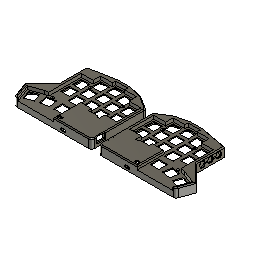
top_23332_3 (Autodesk Fusion 360 design; units mm, degrees)
Autodesk Fusion 360 part; units mm, degrees
sketch "case_plate_23332_3" plane through (0, 0, 0) normal (0, 0, 1) x (1, 0, 0)
  line L0 (107.5, 54.6647) -> (107.5, 98.826)
  line L1 (28.1017, 101.4312) -> (8.5, 89.0512)
  line L2 (107.5, 98.826) -> (67.6888, 106.482)
  line L3 (8.5, 89.0512) -> (8.5, 7.28)
  line L4 (67.5953, 106.5) -> (48.3769, 106.5)
  line L5 (126.2948, 7.28) -> (133.9348, 28.2707)
  line L6 (8.5, 7.28) -> (126.2948, 7.28)
  line L7 (67.6888, 106.482) -> (67.5953, 106.5)
  line L8 (48.3769, 106.5) -> (28.1017, 101.4312)
  line L9 (133.9348, 28.2707) -> (107.5, 54.6647)
  line L10 (48.0076, 109.5) -> (26.9069, 104.2248)
  line L11 (110.5, 101.3041) -> (67.8811, 109.5)
  line L12 (5.5, 90.7047) -> (5.5, 4.28)
  line L13 (128.3954, 4.28) -> (137.4081, 29.0421)
  line L14 (137.4081, 29.0421) -> (110.5, 55.9087)
  line L15 (5.5, 4.28) -> (128.3954, 4.28)
  line L16 (67.8811, 109.5) -> (48.0076, 109.5)
  line L17 (110.5, 55.9087) -> (110.5, 101.3041)
  line L18 (26.9069, 104.2248) -> (5.5, 90.7047)
  line L19 (67.7096, 107.7) -> (48.2292, 107.7)
  line L20 (27.6238, 102.5487) -> (7.3, 89.7126)
  line L21 (108.7, 55.1623) -> (108.7, 99.8172)
  line L22 (135.3241, 28.5793) -> (108.7, 55.1623)
  line L23 (7.3, 89.7126) -> (7.3, 6.08)
  line L24 (7.3, 6.08) -> (127.135, 6.08)
  line L25 (48.2292, 107.7) -> (27.6238, 102.5487)
  line L26 (127.135, 6.08) -> (135.3241, 28.5793)
  line L27 (108.7, 99.8172) -> (67.7096, 107.7)
  line L28 (68.0288, 108.2496) -> (67.7668, 108.3)
  line L29 (67.7668, 108.3) -> (48.1553, 108.3)
  line L30 (27.3848, 103.1074) -> (6.7, 90.0433)
  line L31 (6.7, 90.0433) -> (6.7, 5.48)
  line L32 (109.3, 55.4111) -> (109.3, 100.3128)
  line L33 (48.1553, 108.3) -> (27.3848, 103.1074)
  line L34 (136.0188, 28.7336) -> (109.3, 55.4111)
  line L35 (6.7, 5.48) -> (127.5552, 5.48)
  line L36 (127.5552, 5.48) -> (136.0188, 28.7336)
  line L37 (109.3, 100.3128) -> (68.0288, 108.2496)
  circle A0 centre (32, 80.5) radius 2.2
  circle A1 centre (84, 80.5) radius 2.2
  circle A2 centre (100.1356, 36.6759) radius 2.2
  line L38 (10.5, 10.39) -> (43.5, 10.39)
  line L39 (43.5, 28.39) -> (10.5, 28.39)
  line L40 (43.5, 10.39) -> (43.5, 28.39)
  line L41 (10.5, 28.39) -> (10.5, 10.39)
  line L42 (47.025, 13.01) -> (47.025, 7.16)
  line L43 (55.825, 7.16) -> (55.825, 13.01)
  line L44 (55.825, 13.01) -> (47.025, 13.01)
  line L45 (66.825, 12.025) -> (57.825, 12.025)
  line L46 (57.825, 12.025) -> (57.825, 8.525)
  line L47 (57.825, 8.525) -> (66.825, 8.525)
  line L48 (66.825, 8.525) -> (66.825, 12.025)
  line L49 (122.6064, 37.8282) -> (114.8282, 45.6064)
  line L50 (114.8282, 45.6064) -> (108.3936, 39.1718)
  line L51 (108.3936, 39.1718) -> (110.7259, 36.8394)
  line L52 (118.9049, 34.1268) -> (122.6064, 37.8282)
  line L53 (43.2, 31.55) -> (43.2, 40.45)
  line L54 (43.2, 40.45) -> (35.1996, 40.45)
  line L55 (34.6, 39.7287) -> (34.6, 31.55)
  line L56 (34.6, 31.55) -> (43.2, 31.55)
  line L57 (27, 52) -> (27, 66)
  line L58 (13, 52) -> (27, 52)
  line L59 (13, 66) -> (13, 52)
  line L60 (27, 66) -> (13, 66)
  line L61 (27, 71) -> (27, 85)
  line L62 (13, 85) -> (13, 71)
  line L63 (13, 71) -> (27, 71)
  line L64 (27, 85) -> (13, 85)
  line L65 (46, 59) -> (32, 59)
  line L66 (46, 45) -> (46, 59)
  line L67 (32, 45) -> (46, 45)
  line L68 (32, 59) -> (32, 45)
  line L69 (32, 78) -> (32, 64)
  line L70 (46, 64) -> (46, 78)
  line L71 (32, 64) -> (46, 64)
  line L72 (46, 78) -> (32, 78)
  line L73 (46, 97) -> (32, 97)
  line L74 (32, 83) -> (46, 83)
  line L75 (46, 83) -> (46, 97)
  line L76 (32, 97) -> (32, 83)
  line L77 (51, 64) -> (51, 50)
  line L78 (51, 50) -> (65, 50)
  line L79 (65, 50) -> (65, 64)
  line L80 (65, 64) -> (51, 64)
  line L81 (65, 69) -> (65, 83)
  line L82 (65, 83) -> (51, 83)
  line L83 (51, 83) -> (51, 69)
  line L84 (51, 69) -> (65, 69)
  line L85 (65, 102) -> (51, 102)
  line L86 (51, 102) -> (51, 88)
  line L87 (65, 88) -> (65, 102)
  line L88 (51, 88) -> (65, 88)
  line L89 (84, 59) -> (70, 59)
  line L90 (70, 59) -> (70, 45)
  line L91 (70, 45) -> (84, 45)
  line L92 (84, 45) -> (84, 59)
  line L93 (84, 64) -> (84, 78)
  line L94 (70, 78) -> (70, 64)
  line L95 (84, 78) -> (70, 78)
  line L96 (70, 64) -> (84, 64)
  line L97 (70, 83) -> (84, 83)
  line L98 (70, 97) -> (70, 83)
  line L99 (84, 83) -> (84, 97)
  line L100 (84, 97) -> (70, 97)
  line L101 (89, 66) -> (89, 52)
  line L102 (103, 52) -> (103, 66)
  line L103 (103, 66) -> (89, 66)
  line L104 (89, 52) -> (103, 52)
  line L105 (103, 85) -> (89, 85)
  line L106 (103, 71) -> (103, 85)
  line L107 (89, 85) -> (89, 71)
  line L108 (89, 71) -> (103, 71)
  line L109 (70, 36.2) -> (70, 22.2)
  line L110 (84, 36.2) -> (70, 36.2)
  line L111 (70, 22.2) -> (84, 22.2)
  line L112 (84, 22.2) -> (84, 36.2)
  line L113 (104.164, 19.211) -> (106.5951, 32.9983)
  line L114 (106.5951, 32.9983) -> (92.8078, 35.4294)
  line L115 (92.8078, 35.4294) -> (90.3767, 21.6421)
  line L116 (90.3767, 21.6421) -> (104.164, 19.211)
  line L117 (110.347, 17.5543) -> (123.5027, 12.766)
  line L118 (115.1353, 30.71) -> (110.347, 17.5543)
  line L119 (123.5027, 12.766) -> (128.291, 25.9217)
  line L120 (128.291, 25.9217) -> (115.1353, 30.71)
  line L121 (8.5, 49.25) -> (29.25, 49.25)
  line L122 (10.25, 49.25) -> (10.25, 87.75)
  line L123 (29.25, 87.75) -> (10.25, 87.75)
  line L124 (48.75, 42.25) -> (48.75, 47.25)
  line L125 (29.25, 49.25) -> (29.25, 42.25)
  line L126 (48.25, 99.75) -> (29.25, 99.75)
  line L127 (29.25, 99.75) -> (29.25, 87.75)
  line L128 (48.75, 47.25) -> (67.25, 47.25)
  line L129 (67.75, 99.75) -> (67.75, 104.75)
  line L130 (67.75, 104.75) -> (48.25, 104.75)
  line L131 (48.25, 104.75) -> (48.25, 99.75)
  line L132 (67.25, 4.28) -> (67.25, 47.25)
  line L133 (86.75, 87.75) -> (86.75, 99.75)
  line L134 (86.75, 99.75) -> (67.75, 99.75)
  line L135 (105.75, 54.6647) -> (105.75, 87.75)
  line L136 (105.75, 87.75) -> (86.75, 87.75)
  line L137 (67.25, 19.45) -> (86.9722, 19.45)
  line L138 (86.9722, 19.45) -> (106.6135, 15.9867)
  line L139 (105.75, 35.9398) -> (111.608, 34.9069)
  line L140 (106.6135, 15.9867) -> (125.1463, 9.2413)
  line L141 (123.3406, 4.28) -> (131.8157, 27.5653)
  line L142 (111.7483, 34.8693) -> (133.4723, 26.9624)
  line L143 (105.75, 54.6647) -> (107.5, 54.6647)
  line L144 (111.7483, 34.8693) -> (111.608, 34.9069)
  arc A3 (32, 40.3) -> (34.1857, 42.25) centre (32, 42.5) ccw
  line L145 (34.1857, 42.25) -> (48.75, 42.25)
  line L146 (32, 40.3) -> (29.25, 40.3)
  line L147 (29.25, 42.25) -> (29.25, 40.3)
  line L148 (105.75, 35.9398) -> (105.75, 54.6647)
  line L149 (107.5, 37.4082) -> (107.5, 54.6647)
  line L150 (107.5, 37.4082) -> (111.9871, 36.617)
  line L151 (112.275, 36.5399) -> (111.9871, 36.617)
  line L152 (112.275, 36.5399) -> (133.327, 28.8776)
  line L153 (8.5, 47.65) -> (27.65, 47.65)
  line L154 (27.65, 47.65) -> (27.65, 42.25)
  line L155 (27.65, 42.25) -> (27.65, 38.7)
  line L156 (32, 38.7) -> (27.65, 38.7)
  arc A4 (32, 38.7) -> (35.3193, 40.65) centre (32, 42.5) ccw
  line L157 (35.3193, 40.65) -> (50.35, 40.65)
  line L158 (50.35, 40.65) -> (50.35, 45.65)
  line L159 (50.35, 45.65) -> (65.65, 45.65)
  line L160 (65.65, 4.28) -> (65.65, 45.65)
extrude "Extrude1" add sketch "case_plate_23332_3" against normal blind 7.6 contours L15 L35 L132 L141 | L10 L11 L12 L13 L14 L15 L16 L17 L18 L28 L29 L30 L31 L32 L33 L34 L35 L36 L37 L141 L160 | L15 L35 L132 L160 makes body 1
extrude "Extrude2" add sketch "case_plate_23332_3" against normal blind 6.8 contours L0 L1 L2 L3 L4 L5 L6 L7 L8 L9 L19 L20 L21 L22 L23 L24 L25 L26 L27 L141 L160 | L6 L24 L132 L141 | L6 L24 L132 L160 | L24 L35 L132 L141 | L19 L20 L21 L22 L23 L24 L25 L26 L27 L28 L29 L30 L31 L32 L33 L34 L35 L36 L37 L141 L160 | L24 L35 L132 L160 bodies 1
extrude "Extrude3" add sketch "case_plate_23332_3" along normal blind 7 contours L0 L1 L2 L3 L4 L7 L8 L121 L122 L123 L126 L127 L129 L130 L131 L133 L134 L135 L136 L143 | L0 L1 L2 L3 L4 L5 L6 L7 L8 L9 L19 L20 L21 L22 L23 L24 L25 L26 L27 L141 L160 | L5 L9 L139 L142 L143 L144 L148 L149 L150 L151 L152 | L5 L6 L141 L142 | L6 L24 L132 L160 | L3 L6 L45 L47 L48 L121 L124 L125 L128 L132 A3 L145 L146 L147 L153 L154 L155 L156 A4 L157 L158 L159 L160 | L19 L20 L21 L22 L23 L24 L25 L26 L27 L28 L29 L30 L31 L32 L33 L34 L35 L36 L37 L141 L160 | L24 L35 L132 L160 | L10 L11 L12 L13 L14 L15 L16 L17 L18 L28 L29 L30 L31 L32 L33 L34 L35 L36 L37 L141 L160 | L45 L47 L48 L160 | L15 L35 L132 L160 bodies 1
extrude "Extrude4" add sketch "case_plate_23332_3" along normal blind 1.6 contours L121 L122 L123 L124 L125 L126 L127 L128 L129 L130 L131 L132 L133 L134 L135 L136 L137 L138 L139 L140 L141 L142 L144 A3 L145 L146 L147 L148 | L6 L24 L132 L141 | L6 L132 L137 L138 L140 L141 | L24 L35 L132 L141 | L15 L35 L132 L141 | A0 | A1 | A2 bodies 1
extrude "Extrude5" add sketch "case_plate_23332_3" along normal blind 1.6 from surface at 5.4 contours L9 L49 L50 L51 L52 L149 L150 L152 | L49 L50 L51 L52 L150 L151 L152 | L3 L6 L42 L43 L44 L45 L46 L47 L53 L54 L55 L56 L153 L154 L155 L156 A4 L157 L158 L159 L160 | L6 L42 L43 L44 | L45 L46 L47 L160 | L53 L54 L55 L56 A4 | L38 L39 L40 L41 bodies 1
move_body "Move1" bodies 1 to x (1, 0, 0) y (0, 1, 0) z (0, 0, 1) at (0, 0, -1.6)
hole "Hole1" at (32, 80.5, 0) at (32, 42.5, 0) at (84, 80.5, 0) at (100.1356, 36.6759, 0) direction (0, 0, -1) diameter 2.4 depth 10 tip angle 118 countersink diameter 4.4 countersink angle 90 bodies 1
sketch "Sketch2" plane through (5.5, 0, 0) normal (-1, 0, 0) x (0, -1, 0)
  line L0 (-90.7047, 5.4) -> (-90.7047, -9.2)
  line L1 (-90.7047, -9.2) -> (-4.28, -9.2)
  line L2 (-4.28, -9.2) -> (-4.28, 5.4)
  line L3 (-4.28, 5.4) -> (-90.7047, 5.4)
  line L4 (-28.39, 0) -> (-10.39, 0)
  line L5 (-30.3566, 4.2) -> (-8.4131, 4.2)
  line L6 (-30.3566, -3.8) -> (-7.9707, -3.8)
  line L7 (-25.39, 4.2) -> (-25.39, -3.8)
  line L8 (-13.39, 4.2) -> (-13.39, -3.8)
  dimension "d17" = 1.2
  dimension "d18" = 8
  dimension "d19" = 3
  dimension "d20" = 12
  constraint perpendicular L2 L5
  constraint horizontal L6
  constraint coincident L5 L7.start
  constraint coincident L6 L7.end
  constraint perpendicular L6 L7
  constraint coincident L5 L8.start
  constraint coincident L6 L8.end
  constraint perpendicular L6 L8
  measures "d17" distance of L3 L5
  measures "d18" distance of L5 L6
  measures "d19" distance of L4.start L7
  measures "d20" distance of L7 L8
extrude "Extrude6" cut sketch "Sketch2" against normal up to surface (3 mm away) contours L4 L5 L7 L8 | L4 L6 L7 L8 bodies 1
chamfer "Chamfer2" distance 1 angle 45 4 edges at (5.5, 19.39, 4.2) (5.5, 25.39, 0.2) (5.5, 19.39, -3.8) (5.5, 13.39, 0.2) on bodies 1
sketch "Sketch3" plane through (0, 4.28, 0) normal (0, -1, 0) x (1, 0, 0)
  line L0 (5.5, 5.4) -> (5.5, -9.2)
  line L1 (5.5, -9.2) -> (128.3954, -9.2)
  line L2 (128.3954, -9.2) -> (128.3954, 5.4)
  line L3 (128.3954, 5.4) -> (123.3406, 5.4)
  line L4 (123.3406, 5.4) -> (123.3406, 0)
  line L5 (123.3406, 0) -> (67.25, 0)
  line L6 (67.25, 0) -> (67.25, 5.4)
  line L7 (67.25, 5.4) -> (5.5, 5.4)
  line L8 (55.825, 0) -> (47.025, 0)
  line L9 (46.3828, -5) -> (57.0469, -5) construction
  line L10 (46.1538, -4.25) -> (57.6357, -4.25) construction
  line L11 (49.425, 0) -> (49.425, -4.25) construction
  line L12 (53.425, 0) -> (53.425, -4.25) construction
  line L13 (49.425, -5.75) -> (53.425, -5.75)
  arc A0 (53.425, -5.75) -> (53.425, -2.75) centre (53.425, -4.25) ccw
  line L14 (53.425, -2.75) -> (49.425, -2.75)
  arc A1 (49.425, -2.75) -> (49.425, -5.75) centre (49.425, -4.25) ccw
  line L15 (49.425, -4.25) -> (53.425, -4.25) construction
  dimension "d23" = 10.4
  dimension "d24" = 0.75
  dimension "d25" = 2.4
  dimension "d26" = 4
  dimension "d27" = 3
  constraint horizontal L9
  constraint parallel L9 L10
  constraint coincident L8 L11.start
  constraint coincident L10 L11.end
  constraint perpendicular L10 L11
  constraint coincident L8 L12.start
  constraint coincident L10 L12.end
  constraint perpendicular L10 L12
  constraint tangent L13 A0
  constraint tangent A0 L14
  constraint parallel L13 L14
  constraint tangent L14 A1
  constraint tangent L13 A1
  constraint coincident L12.end A0.centre
  constraint perpendicular L12 L15
  constraint coincident L11.end A1.centre
  measures "d23" distance of L7 L9
  measures "d24" distance of L9 L10
  measures "d25" distance of L8.end L11
  measures "d26" distance of L11 L12
  measures "d27" diameter of A0
extrude "Extrude7" cut sketch "Sketch3" against normal up to surface (3 mm away) contours L13 A0 L14 A1 bodies 1
sketch "Sketch4" plane through (0, 0, -5.75) normal (0, 0, 1) x (-1, 0, 0)
  line L0 (-49.425, -4.28) -> (-53.425, -4.28)
  line L1 (-53.425, -4.28) -> (-53.425, -7.28)
  line L2 (-53.425, -7.28) -> (-49.425, -7.28)
  line L3 (-49.425, -7.28) -> (-49.425, -4.28)
  line L4 (-49.425, -5.78) -> (-53.425, -5.78)
  constraint midpoint L3 L4.start
  constraint midpoint L1 L4.end
extrude "Extrude8" cut sketch "Sketch4" against normal up to surface (2.65 mm away) contours L1 L2 L3 L4 bodies 1
chamfer "Chamfer1" distance 0.5 angle 45 4 edges at (51.425, 4.28, -2.75) (54.925, 4.28, -4.25) (51.425, 4.28, -5.75) (47.925, 4.28, -4.25) on bodies 1
sketch "Sketch5" plane through (83.1189, 83.2475, 0) normal (0.70656, 0.707653, 0) x (-0.707653, 0.70656, 0)
  line L0 (-76.7172, 5.4) -> (-76.7172, -9.2)
  line L1 (-76.7172, -9.2) -> (-38.6928, -9.2)
  line L2 (-38.6928, -9.2) -> (-38.6928, 5.4)
  line L3 (-38.6928, 5.4) -> (-76.7172, 5.4)
  line L4 (-76.7172, -5) -> (-38.6928, -5) construction
  line L5 (-60.0349, 0) -> (-49.0349, 0) construction
  line L6 (-58.0349, -3.1835) -> (-58.0349, -6.8453)
  line L7 (-51.0349, -3.1591) -> (-51.0349, -7.1366)
  line L8 (-58.0349, -4.5) -> (-51.0349, -4.5)
  line L9 (-58.0349, -5.5) -> (-51.0349, -5.5)
  dimension "d34" = 10.4
  dimension "d35" = 2
  dimension "d36" = 7
  dimension "d37" = 0.5
  dimension "d38" = 0.5
  constraint coincident L0 L4.start
  constraint coincident L2 L4.end
  constraint perpendicular L2 L4
  constraint perpendicular L4 L6
  constraint perpendicular L4 L7
  constraint coincident L6 L8.start
  constraint coincident L7 L8.end
  constraint perpendicular L7 L8
  constraint coincident L6 L9.start
  constraint coincident L7 L9.end
  constraint perpendicular L7 L9
  measures "d34" distance of L3 L4
  measures "d35" distance of L5.start L6
  measures "d36" distance of L6 L7
  measures "d37" distance of L4 L9
  measures "d38" distance of L4 L8
extrude "Extrude9" cut sketch "Sketch5" against normal up to surface (3 mm away) contours L6 L7 L8 L9 bodies 1
sketch "Sketch6" plane through (0, 0, 5.4) normal (0, 0, 1) x (-1, 0, 0)
  line L0 (-111.7483, -34.8693) -> (-131.8157, -27.5653)
  line L1 (-131.8157, -27.5653) -> (-123.3406, -4.28)
  line L2 (-123.3406, -4.28) -> (-128.3954, -4.28)
  line L3 (-128.3954, -4.28) -> (-137.4081, -29.0421)
  line L4 (-137.4081, -29.0421) -> (-110.5, -55.9087)
  line L5 (-110.5, -55.9087) -> (-110.5, -101.3041)
  line L6 (-110.5, -101.3041) -> (-67.8811, -109.5)
  line L7 (-67.8811, -109.5) -> (-48.0076, -109.5)
  line L8 (-48.0076, -109.5) -> (-26.9069, -104.2248)
  line L9 (-26.9069, -104.2248) -> (-5.5, -90.7047)
  line L10 (-5.5, -90.7047) -> (-5.5, -4.28)
  line L11 (-5.5, -4.28) -> (-67.25, -4.28)
  line L12 (-67.25, -4.28) -> (-67.25, -47.25)
  line L13 (-67.25, -47.25) -> (-48.75, -47.25)
  line L14 (-48.75, -47.25) -> (-48.75, -42.25)
  line L15 (-48.75, -42.25) -> (-34.1857, -42.25)
  arc A0 (-32, -40.3) -> (-34.1857, -42.25) centre (-32, -42.5) ccw
  line L16 (-32, -40.3) -> (-29.25, -40.3)
  line L17 (-29.25, -40.3) -> (-29.25, -49.25)
  line L18 (-29.25, -49.25) -> (-10.25, -49.25)
  line L19 (-10.25, -49.25) -> (-10.25, -87.75)
  line L20 (-10.25, -87.75) -> (-29.25, -87.75)
  line L21 (-29.25, -87.75) -> (-29.25, -99.75)
  line L22 (-29.25, -99.75) -> (-48.25, -99.75)
  line L23 (-48.25, -99.75) -> (-48.25, -104.75)
  line L24 (-48.25, -104.75) -> (-67.75, -104.75)
  line L25 (-67.75, -104.75) -> (-67.75, -99.75)
  line L26 (-67.75, -99.75) -> (-86.75, -99.75)
  line L27 (-86.75, -99.75) -> (-86.75, -87.75)
  line L28 (-86.75, -87.75) -> (-105.75, -87.75)
  line L29 (-105.75, -87.75) -> (-105.75, -35.9398)
  line L30 (-105.75, -35.9398) -> (-111.608, -34.9069)
  line L31 (-111.608, -34.9069) -> (-111.7483, -34.8693)
  line L32 (-66.825, -12.025) -> (-57.825, -12.025)
  line L33 (-57.825, -12.025) -> (-57.825, -8.525)
  line L34 (-57.825, -8.525) -> (-66.825, -8.525)
  line L35 (-66.825, -8.525) -> (-66.825, -12.025)
  line L36 (-59.325, -12.025) -> (-59.325, -8.525)
  line L37 (-65.325, -12.025) -> (-65.325, -8.525)
  dimension "d41" = 1.5
  dimension "d42" = 6
  constraint coincident L32 L36.start
  constraint coincident L34 L36.end
  constraint perpendicular L34 L36
  constraint coincident L32 L37.start
  constraint coincident L34 L37.end
  constraint perpendicular L34 L37
  measures "d41" distance of L33 L36
  measures "d42" distance of L36 L37
extrude "Extrude10" cut sketch "Sketch6" against normal up to surface (1.6 mm away) contours L32 L34 L36 L37 bodies 1
chamfer "Chamfer3" distance 0.4 angle 45 4 edges at (62.325, 12.025, 5.4) (59.325, 10.275, 5.4) (62.325, 8.525, 5.4) (65.325, 10.275, 5.4) on bodies 1
sketch "Sketch7" plane through (110.5, 0, 0) normal (1, 0, 0) x (0, 1, 0)
  line L0 (55.9087, 5.4) -> (55.9087, -9.2)
  line L1 (55.9087, -9.2) -> (101.3041, -9.2)
  line L2 (101.3041, -9.2) -> (101.3041, 5.4)
  line L3 (101.3041, 5.4) -> (55.9087, 5.4)
  line L4 (55.9087, -1.5) -> (101.3041, -1.5) construction
  line L5 (67.8782, 2.4883) -> (63.2884, 2.4616)
  line L6 (63.2884, 2.4616) -> (61.0165, -1.5266)
  line L7 (61.0165, -1.5266) -> (63.3345, -5.4883)
  line L8 (63.3345, -5.4883) -> (67.9244, -5.4616)
  line L9 (67.9244, -5.4616) -> (70.1962, -1.4734)
  line L10 (70.1962, -1.4734) -> (67.8782, 2.4883)
  line L11 (80.8782, 2.4883) -> (76.2884, 2.4616)
  line L12 (76.2884, 2.4616) -> (74.0165, -1.5266)
  line L13 (74.0165, -1.5266) -> (76.3345, -5.4883)
  line L14 (76.3345, -5.4883) -> (80.9244, -5.4616)
  line L15 (80.9244, -5.4616) -> (83.1962, -1.4734)
  line L16 (83.1962, -1.4734) -> (80.8782, 2.4883)
  line L17 (93.8782, 2.4883) -> (89.2884, 2.4616)
  line L18 (89.2884, 2.4616) -> (87.0165, -1.5266)
  line L19 (87.0165, -1.5266) -> (89.3345, -5.4883)
  line L20 (89.3345, -5.4883) -> (93.9244, -5.4616)
  line L21 (93.9244, -5.4616) -> (96.1962, -1.4734)
  line L22 (96.1962, -1.4734) -> (93.8782, 2.4883)
  line L23 (65.6064, -2.25) -> (91.6064, -2.25)
  arc A0 (91.6064, -2.25) -> (91.6064, -0.75) centre (91.6064, -1.5) ccw
  line L24 (91.6064, -0.75) -> (65.6064, -0.75)
  arc A1 (65.6064, -0.75) -> (65.6064, -2.25) centre (65.6064, -1.5) ccw
  line L25 (65.6064, -1.5) -> (91.6064, -1.5) construction
  point P0 (78.6064, -1.5)
  point P1 (91.6064, -1.5)
  point P2 (65.6064, -1.5)
  point P3 (65.6064, -1.5)
  point P4 (78.6064, -1.5)
  point P5 (91.6064, -1.5)
  dimension "d46" = 6.9
  dimension "d47" = 13
  dimension "d48" = 13
  dimension "d49" = 3.975
  dimension "d50" = 3.975
  dimension "d51" = 3.975
  dimension "d52" = 1.5
  constraint coincident L0 L4.start
  constraint coincident L2 L4.end
  constraint perpendicular L2 L4
  constraint midpoint L4 P4
  constraint coincident L4 P5
  constraint coincident L4 P3
  constraint coincident P3 P2
  constraint coincident P4 P0
  constraint coincident P5 P1
  constraint tangent L23 A0
  constraint tangent A0 L24
  constraint parallel L23 L24
  constraint tangent L24 A1
  constraint tangent L23 A1
  constraint parallel L4 L25
  measures "d46" distance of L3 L4
  measures "d47" distance of P4 P3
  measures "d48" distance of P4 P5
  measures "d49" distance of P3 L10
  measures "d50" distance of P4 L16
  measures "d51" distance of P5 L22
  measures "d52" diameter of A0
extrude "Extrude11" cut sketch "Sketch7" against normal blind 2 contours L5 L6 L7 L8 L9 L10 L23 L24 A1 | L9 L10 L12 L13 L23 L24 | L9 L10 L23 L24 A1 | L12 L13 L15 L16 L23 L24 | L11 L12 L16 L24 | L15 L16 L18 L19 L23 L24 | L13 L14 L15 L23 | L18 L19 L23 A0 L24 | L17 L18 L19 L20 L21 L22 L23 A0 L24 bodies 1
sketch "Sketch8" plane through (83.1189, 83.2475, 0) normal (0.70656, 0.707653, 0) x (-0.707653, 0.70656, 0)
  line L0 (-58.0349, -4.5) -> (-51.0349, -4.5)
  line L1 (-51.0349, -4.5) -> (-51.0349, -5.5)
  line L2 (-51.0349, -5.5) -> (-58.0349, -5.5)
  line L3 (-58.0349, -5.5) -> (-58.0349, -4.5)
  line L4 (-76.7172, 5.4) -> (-76.7172, -9.2)
  line L5 (-76.7172, -9.2) -> (-38.6928, -9.2)
  line L6 (-38.6928, -9.2) -> (-38.6928, 5.4)
  line L7 (-38.6928, 5.4) -> (-76.7172, 5.4)
  line L8 (-76.7172, -1.5) -> (-38.6928, -1.5) construction
  line L9 (-62.4117, 2.4689) -> (-67.0017, 2.4811)
  line L10 (-67.0017, 2.4811) -> (-69.3071, -1.4879)
  line L11 (-69.3071, -1.4879) -> (-67.0227, -5.4689)
  line L12 (-67.0227, -5.4689) -> (-62.4328, -5.4811)
  line L13 (-62.4328, -5.4811) -> (-60.1273, -1.5121)
  line L14 (-60.1273, -1.5121) -> (-62.4117, 2.4689)
  line L15 (-51.2827, -1.5121) -> (-48.9773, -5.4811)
  line L16 (-48.9773, -5.4811) -> (-44.3873, -5.4689)
  line L17 (-44.3873, -5.4689) -> (-42.1029, -1.4879)
  line L18 (-42.1029, -1.4879) -> (-44.4084, 2.4811)
  line L19 (-44.4084, 2.4811) -> (-48.9983, 2.4689)
  line L20 (-48.9983, 2.4689) -> (-51.2827, -1.5121)
  line L21 (-64.7172, -2.25) -> (-46.6928, -2.25)
  arc A0 (-46.6928, -2.25) -> (-46.6928, -0.75) centre (-46.6928, -1.5) ccw
  line L22 (-46.6928, -0.75) -> (-64.7172, -0.75)
  arc A1 (-64.7172, -0.75) -> (-64.7172, -2.25) centre (-64.7172, -1.5) ccw
  line L23 (-64.7172, -1.5) -> (-46.6928, -1.5) construction
  point P0 (-64.7172, -1.5)
  point P1 (-46.6928, -1.5)
  point P2 (-64.7172, -1.5)
  point P3 (-46.6928, -1.5)
  dimension "d55" = 6.9
  dimension "d56" = 8
  dimension "d57" = 12
  dimension "d58" = 3.975
  dimension "d59" = 3.975
  dimension "d60" = 1.5
  constraint coincident L4 L8.start
  constraint coincident L6 L8.end
  constraint perpendicular L6 L8
  constraint coincident L8 P2
  constraint coincident L8 P3
  constraint coincident P2 P0
  constraint coincident P3 P1
  constraint tangent L21 A0
  constraint tangent A0 L22
  constraint parallel L21 L22
  constraint tangent L22 A1
  constraint tangent L21 A1
  constraint parallel L8 L23
  measures "d55" distance of L7 L8
  measures "d56" distance of L6 P3
  measures "d57" distance of L4 P2
  measures "d58" distance of P2 L14
  measures "d59" distance of P3 L20
  measures "d60" diameter of A0
extrude "Extrude12" cut sketch "Sketch8" against normal blind 2 contours L9 L10 L11 L12 L13 L14 L21 L22 A1 | L13 L14 L15 L20 L21 L22 | L13 L14 L21 L22 A1 | L15 L20 L21 A0 L22 | L15 L16 L17 L18 L19 L20 L21 A0 L22 bodies 1
chamfer "Chamfer4" distance 0.4 angle 45 30 edges at (131.3486, 35.0923, 0.4966) (131.356, 35.0849, -3.4784) (128.9237, 37.5134, -5.475) (126.6356, 39.798, -3.8655) (126.6312, 39.8024, 0.8595) (128.9088, 37.5283, 2.475) (118.4463, 47.9747, 0.8595) (118.4419, 47.979, -3.8655) (116.1538, 50.2636, -5.475) (113.7214, 52.6922, -3.4784) (113.7289, 52.6848, 0.4966) (116.1687, 50.2488, 2.475) (110.5, 62.1524, 0.4675) (110.5, 62.1755, -3.5074) (110.5, 65.6294, -5.4749) (110.5, 68.8391, -3.8558) (110.5, 68.8256, 0.8691) (110.5, 65.5833, 2.4749) (110.5, 75.3736, 0.8558) (110.5, 75.3871, -3.8691) (110.5, 78.6294, -5.4749) (110.5, 81.8391, -3.8558) (110.5, 81.8256, 0.8691) (110.5, 78.5833, 2.4749) (110.5, 88.3736, 0.8558) (110.5, 91.5833, 2.4749) (110.5, 88.3871, -3.8691) (110.5, 91.6294, -5.4749) (110.5, 95.0603, -3.4675) (110.5, 95.0372, 0.5074) on bodies 1
fillet "Fillet1" radius 5 12 edges at (128.3954, 4.28, -1.9) (5.5, 4.28, -1.9) (5.5, 90.7047, -1.9) (26.9069, 104.2248, -1.9) (67.8811, 109.5, -1.9) (48.0076, 109.5, -1.9) (127.5552, 5.48, -8.8) (6.7, 5.48, -8.8) (6.7, 90.0433, -8.8) (27.3848, 103.1074, -8.8) (48.1553, 108.3, -8.8) (67.7668, 108.3, -8.8) on bodies 1
fillet "Fillet1" radius 2 6 edges at (67.5953, 106.5, -5) (48.3769, 106.5, -5) (28.1017, 101.4312, -5) (8.5, 89.0512, -5) (8.5, 7.28, -2.3) (126.2948, 7.28, -5) on bodies 1
chamfer "Chamfer5" distance 1.5 angle 45 18 edges at (67.25, 25.765, 5.4) (38.875, 4.28, 5.4) (89.4245, 105.357, 5.4) (67.879, 109.4775, 5.4) (58.0139, 109.5, 5.4) (48.0122, 109.4625, 5.4) (37.548, 106.8851, 5.4) (26.9321, 104.166, 5.4) (17.0292, 97.9863, 5.4) (6.1211, 90.3624, 5.4) (5.5, 48.6144, 5.4) (6.9645, 5.7445, 5.4) (110.5, 78.6064, 5.4) (123.954, 42.4754, 5.4) (133.5005, 18.306, 5.4) (124.1175, 4.28, 5.4) (127.7623, 5.1843, 5.4) (127.5781, 15.9227, 5.4) on bodies 1
mirror "Mirror1" about plane through (0, 0, 0) normal (1, 0, 0) of bodies 1 makes body 2
